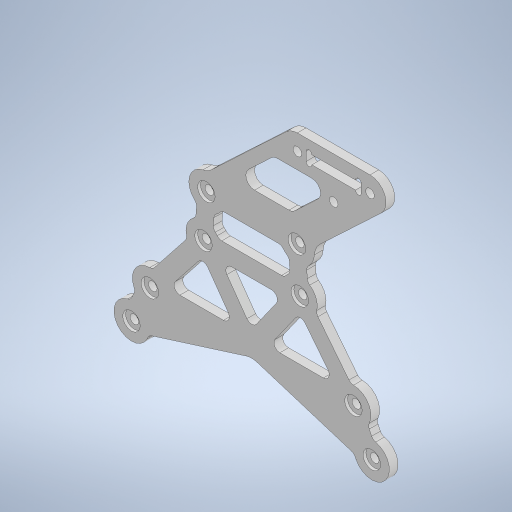
# Autodesk Inventor part: 外中間ユニット
Saved by Autodesk Inventor 2023 (Build 270158000, 158)
## iProperties
Created: 2022-06-23
Part Number: 外中間ユニット
Material: 一般
Document SubType Name: Modeling
Designer: muzho
Density: 1 g/cm^3
Appearance: 既定
Author: muzho
Autodesk Inventor part; units mm, degrees
ref_plane "YZ Plane" through (0, 0, 0) normal (1, 0, 0) x (0, 1, 0)
ref_plane "XZ Plane" through (0, 0, 0) normal (0, 1, 0) x (-1, 0, 0)
ref_plane "XY Plane" through (0, 0, 0) normal (0, 0, 1) x (1, 0, 0)
sketch "スケッチ1" plane through (0, 0, 0) normal (0, 0, 1) x (1, 0, 0)
  line L0 (35.7118, 64.4865) -> (20.7118, 64.4865)
  arc A0 (18.7118, 64.4865) -> (20.7118, 64.4865) centre (19.7118, 64.4865) ccw
  line L1 (18.7118, 64.4865) -> (18.7118, 67.4865)
  arc A1 (20.7118, 67.4865) -> (18.7118, 67.4865) centre (19.7118, 67.4865) ccw
  line L2 (20.7118, 67.4865) -> (35.7118, 67.4865)
  arc A2 (37.7118, 67.4865) -> (35.7118, 67.4865) centre (36.7118, 67.4865) ccw
  line L3 (37.7118, 67.4865) -> (37.7118, 64.4865)
  arc A3 (35.7118, 64.4865) -> (37.7118, 64.4865) centre (36.7118, 64.4865) ccw
  line L4 (8.8657, 60.4865) -> (20.7172, 60.4865)
  arc A4 (22.7728, 55.3014) -> (20.7172, 60.4865) centre (20.7172, 57.4865) ccw
  line L5 (22.7728, 55.3014) -> (14.8948, 47.89)
  arc A5 (12.8392, 47.0751) -> (14.8948, 47.89) centre (12.8392, 50.0751) ccw
  line L6 (12.8392, 47.0751) -> (0.9877, 47.0751)
  arc A6 (-1.0679, 52.2601) -> (0.9877, 47.0751) centre (0.9877, 50.0751) ccw
  line L7 (-1.0679, 52.2601) -> (6.8101, 59.6715)
  arc A7 (8.8657, 60.4865) -> (6.8101, 59.6715) centre (8.8657, 57.4865) ccw
  circle A8 centre (40.7118, 65.9865) radius 1.5
  circle A9 centre (28.2118, 57.2015) radius 1.5
  circle A10 centre (15.7118, 65.9865) radius 1.5
  circle A11 centre (41.3199, -13) radius 1.5
  circle A12 centre (-35, 0) radius 1.5
  circle A13 centre (-16.5506, 23.3453) radius 1.5
  circle A14 centre (35, 0) radius 1.5
  circle A15 centre (15.5646, 38.363) radius 1.5
  circle A16 centre (-41.3199, -13) radius 1.5
  circle A17 centre (-15.5646, 38.363) radius 1.5
  circle A18 centre (16.5506, 23.3453) radius 1.5
  line L8 (-1.8007, -3.7115) -> (-34.3942, -13.966)
  arc A19 (1.8007, -3.7115) -> (-1.8007, -3.7115) centre (0, -9.4349) ccw
  line L9 (34.3942, -13.966) -> (1.8007, -3.7115)
  arc A20 (35.5927, -14.9994) -> (34.3942, -13.966) centre (33.794, -15.8738) ccw
  line L10 (35.9013, -15.6342) -> (35.5927, -14.9994)
  arc A21 (35.9013, -15.6342) -> (42.6355, -7.1204) centre (41.3199, -13) ccw
  arc A22 (41.2736, -6.0431) -> (42.6355, -7.1204) centre (43.0723, -5.1687) ccw
  line L11 (40.4425, -4.3336) -> (41.2736, -6.0431)
  arc A23 (40.4365, -2.5971) -> (40.4425, -4.3336) centre (42.2412, -3.4591) ccw
  arc A24 (40.4365, -2.5971) -> (35.0232, 6.025) centre (35, 0) ccw
  arc A25 (33.4618, 6.7849) -> (35.0232, 6.025) centre (35.0309, 8.0249) ccw
  line L12 (22.7963, 20.2807) -> (33.4618, 6.7849)
  arc A26 (22.4178, 21.9755) -> (22.7963, 20.2807) centre (24.3654, 21.5207) ccw
  arc A27 (22.4178, 21.9755) -> (19.9877, 28.2938) centre (16.5506, 23.3453) ccw
  arc A28 (19.1329, 29.8054) -> (19.9877, 28.2938) centre (21.1286, 29.9364) ccw
  line L13 (18.9694, 32.296) -> (19.1329, 29.8054)
  arc A29 (19.6192, 33.9064) -> (18.9694, 32.296) centre (20.9651, 32.4271) ccw
  arc A30 (19.6192, 33.9064) -> (21.584, 38.1019) centre (15.5646, 38.363) ccw
  arc A31 (23.4671, 42.2119) -> (21.584, 38.1019) centre (27.5783, 37.8418) ccw
  line L14 (23.4671, 42.2119) -> (44.4804, 61.9806)
  arc A32 (44.4804, 61.9806) -> (40.7118, 71.4865) centre (40.7118, 65.9865) ccw
  line L15 (40.7118, 71.4865) -> (15.7118, 71.4865)
  arc A33 (15.7118, 71.4865) -> (11.9431, 69.9924) centre (15.7118, 65.9865) ccw
  line L16 (11.9431, 69.9924) -> (-13.7829, 45.7901)
  arc A34 (-16.7318, 44.2739) -> (-13.7829, 45.7901) centre (-17.8942, 50.1602) ccw
  arc A35 (-16.7318, 44.2739) -> (-19.6192, 33.9064) centre (-15.5646, 38.363) ccw
  arc A36 (-18.9694, 32.296) -> (-19.6192, 33.9064) centre (-20.9651, 32.4271) ccw
  line L17 (-19.1329, 29.8054) -> (-18.9694, 32.296)
  arc A37 (-19.9877, 28.2938) -> (-19.1329, 29.8054) centre (-21.1286, 29.9364) ccw
  arc A38 (-19.9877, 28.2938) -> (-22.4178, 21.9755) centre (-16.5506, 23.3453) ccw
  arc A39 (-22.7963, 20.2807) -> (-22.4178, 21.9755) centre (-24.3654, 21.5207) ccw
  line L18 (-33.4618, 6.7849) -> (-22.7963, 20.2807)
  arc A40 (-35.0232, 6.025) -> (-33.4618, 6.7849) centre (-35.0309, 8.0249) ccw
  arc A41 (-35.0232, 6.025) -> (-40.4365, -2.5971) centre (-35, 0) ccw
  arc A42 (-40.4425, -4.3336) -> (-40.4365, -2.5971) centre (-42.2412, -3.4591) ccw
  line L19 (-41.2736, -6.0431) -> (-40.4425, -4.3336)
  arc A43 (-42.6355, -7.1204) -> (-41.2736, -6.0431) centre (-43.0723, -5.1687) ccw
  arc A44 (-42.6355, -7.1204) -> (-35.9013, -15.6342) centre (-41.3199, -13) ccw
  line L20 (-35.5927, -14.9994) -> (-35.9013, -15.6342)
  arc A45 (-34.3942, -13.966) -> (-35.5927, -14.9994) centre (-33.794, -15.8738) ccw
  arc A46 (-13.1458, 29.4123) -> (-12.496, 27.8019) centre (-11.1501, 29.2813) ccw
  line L21 (-12.9823, 31.903) -> (-13.1458, 29.4123)
  arc A47 (-12.1275, 33.4146) -> (-12.9823, 31.903) centre (-10.9866, 31.7719) ccw
  arc A48 (-12.1275, 33.4146) -> (-10.852, 34.6091) centre (-15.5646, 38.363) ccw
  arc A49 (-9.2876, 35.363) -> (-10.852, 34.6091) centre (-9.2876, 33.363) ccw
  line L22 (9.2876, 35.363) -> (-9.2876, 35.363)
  arc A50 (10.852, 34.6091) -> (9.2876, 35.363) centre (9.2876, 33.363) ccw
  arc A51 (10.852, 34.6091) -> (12.1275, 33.4146) centre (15.5646, 38.363) ccw
  arc A52 (12.9823, 31.903) -> (12.1275, 33.4146) centre (10.9866, 31.7719) ccw
  line L23 (13.1458, 29.4123) -> (12.9823, 31.903)
  arc A53 (12.496, 27.8019) -> (13.1458, 29.4123) centre (11.1501, 29.2813) ccw
  arc A54 (12.496, 27.8019) -> (11.838, 27.0992) centre (16.5506, 23.3453) ccw
  arc A55 (10.2736, 26.3453) -> (11.838, 27.0992) centre (10.2736, 28.3453) ccw
  line L24 (-10.2736, 26.3453) -> (10.2736, 26.3453)
  arc A56 (-11.838, 27.0992) -> (-10.2736, 26.3453) centre (-10.2736, 28.3453) ccw
  arc A57 (-11.838, 27.0992) -> (-12.496, 27.8019) centre (-16.5506, 23.3453) ccw
  arc A58 (-15.1362, 16.1631) -> (-18.337, 16.2465) centre (-16.7678, 15.0064) ccw
  line L25 (-8.0422, 6.1567) -> (-15.1362, 16.1631)
  arc A59 (-9.6738, 3) -> (-8.0422, 6.1567) centre (-9.6738, 5) ccw
  line L26 (-24.6757, 3) -> (-9.6738, 3)
  arc A60 (-26.2449, 6.2401) -> (-24.6757, 3) centre (-24.6757, 5) ccw
  line L27 (-18.337, 16.2465) -> (-26.2449, 6.2401)
  arc A61 (8.5084, 17.1886) -> (6.8768, 20.3453) centre (6.8768, 18.3453) ccw
  line L28 (1.6316, 7.4886) -> (8.5084, 17.1886)
  arc A62 (-1.6316, 7.4886) -> (1.6316, 7.4886) centre (0, 8.6453) ccw
  line L29 (-8.5084, 17.1886) -> (-1.6316, 7.4886)
  arc A63 (-6.8768, 20.3453) -> (-8.5084, 17.1886) centre (-6.8768, 18.3453) ccw
  line L30 (6.8768, 20.3453) -> (-6.8768, 20.3453)
  arc A64 (18.337, 16.2465) -> (15.1362, 16.1631) centre (16.7678, 15.0064) ccw
  line L31 (26.2449, 6.2401) -> (18.337, 16.2465)
  arc A65 (24.6757, 3) -> (26.2449, 6.2401) centre (24.6757, 5) ccw
  line L32 (9.6738, 3) -> (24.6757, 3)
  arc A66 (8.0422, 6.1567) -> (9.6738, 3) centre (9.6738, 5) ccw
  line L33 (15.1362, 16.1631) -> (8.0422, 6.1567)
  circle A67 centre (-15.5646, 38.363) radius 3.025
  circle A68 centre (15.5646, 38.363) radius 3.025
  circle A69 centre (-16.5506, 23.3453) radius 3.025
  circle A70 centre (16.5506, 23.3453) radius 3.025
  circle A71 centre (-35, 0) radius 3.025
  circle A72 centre (-41.3199, -13) radius 3.025
  circle A73 centre (35, 0) radius 3.025
  circle A74 centre (41.3199, -13) radius 3.025
  point P0 (0, 0)
  point P1 (0, 0)
  dimension "d0" = 6.05
  dimension "d1" = 6.05
  dimension "d2" = 6.05
  dimension "d3" = 6.05
  dimension "d4" = 6.05
  dimension "d5" = 6.05
  dimension "d6" = 6.05
  dimension "d7" = 6.05
  constraints: 112 point on circle, 75 centre point, 68 end point, 10 horizontal, 8 coincident, 2 vertical, 248 other
  measures "d0" diameter of A67
  measures "d1" diameter of A68
  measures "d2" diameter of A69
  measures "d3" diameter of A70
  measures "d4" diameter of A71
  measures "d5" diameter of A72
  measures "d6" diameter of A73
  measures "d7" diameter of A74
extrude "押し出し1" add sketch "スケッチ1" along normal blind 3 contours L8 A45 L20 A44 A43 L19 A42 A41 A40 L18 A39 A38 A37 L17 A36 A35 A34 L16 A33 L15 A32 L14 A31 A30 A29 L13 A28 A27 A26 L12 A25 A24 A23 L11 A22 A21 L10 A20 L9 A19
extrude "押し出し2" add sketch "スケッチ1" along normal blind 2 contours A67 | A68 | A69 | A70 | A71 | A72 | A73 | A74
